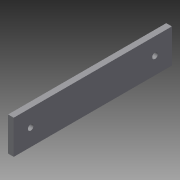
# Autodesk Inventor part: rail supporter plate
Saved by Autodesk Inventor 2015 (Build 190159000, 159)
## iProperties
Created: 2015-01-22
Part Number: rail supporter plate
Material: Generic
Document SubType Name: Modeling
Designer: 215152
Density: 1 g/cm^3
Appearance: Default
Author: 215152
Autodesk Inventor part; units mm, degrees
ref_plane "YZ Plane" through (0, 0, 0) normal (1, 0, 0) x (0, 1, 0)
ref_plane "XZ Plane" through (0, 0, 0) normal (0, 1, 0) x (-1, 0, 0)
ref_plane "XY Plane" through (0, 0, 0) normal (0, 0, 1) x (1, 0, 0)
sketch "Sketch1" plane through (0, 0, 0) normal (1, 0, 0) x (0, 1, 0)
  line L0 (0, 0) -> (-38.1, 0)
  line L1 (-38.1, 0) -> (-38.1, 228.6)
  line L2 (-38.1, 228.6) -> (0, 228.6)
  line L3 (0, 228.6) -> (0, 0)
  circle A0 centre (-19.05, 209.55) radius 3.175
  circle A1 centre (-19.05, 19.05) radius 3.175
  dimension "d0" = 38.1
  dimension "d1" = 228.6
  dimension "d2" = 19.05
  dimension "d3" = 19.05
  dimension "d4" = 19.05
  dimension "d5" = 19.05
  dimension "d6" = 6.35
  dimension "d7" = 6.35
  constraints: 8 end point, 2 centre point, 2 coincident, 2 parallel, 1 horizontal, 1 perpendicular
  measures "d0" distance of L1.end L2.end
  measures "d1" distance of L0.end L1.end
  measures "d2" distance from line of L3 point (-19.05, 209.55)
  measures "d3" distance from line of L2 point (-19.05, 209.55)
  measures "d4" distance from line of L0 point (-19.05, 19.05)
  measures "d5" distance from line of L3 point (-19.05, 19.05)
  measures "d6" diameter of A0
  measures "d7" diameter of A1
extrude "Extrusion1" add sketch "Sketch1" along normal blind 6.35
body "Solid1"
